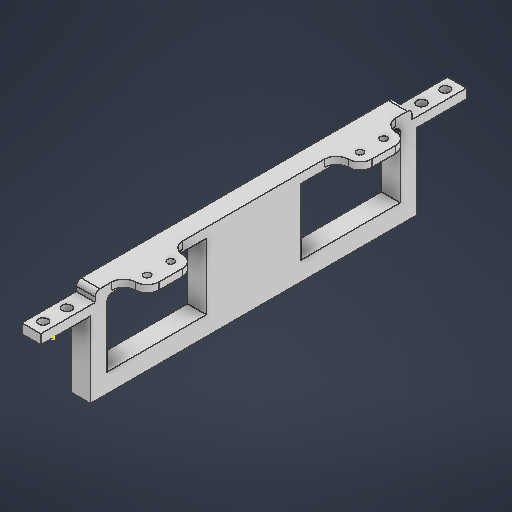
# Autodesk Inventor part: side_wall2
Saved by Autodesk Inventor 2026.1 (Build 301233000, 233)
## iProperties
Created: 2026-03-22
Part Number: side_wall2
Material: Generic
Document SubType Name: Modeling
Designer: emanuel
Density: 1 g/cm^3
Appearance: Default
Author: emanuel
Autodesk Inventor part; units mm, degrees
ref_plane "YZ Plane" through (0, 0, 0) normal (1, 0, 0) x (0, 1, 0)
ref_plane "XZ Plane" through (0, 0, 0) normal (0, 1, 0) x (-1, 0, 0)
ref_plane "XY Plane" through (0, 0, 0) normal (0, 0, 1) x (1, 0, 0)
sketch "Sketch1" plane through (0, 0, 0) normal (0, 1, 0) x (-1, 0, 0)
  circle A0 centre (0, 0) radius 2
  line L0 (0, 0) -> (0, -10)
  circle A1 centre (0, -10) radius 2
  line L1 (0, 0) -> (4, 0)
  line L2 (4, 0) -> (4, 5)
  line L3 (4, 5) -> (0, 5)
  line L4 (0, 5) -> (0, 0)
  line L5 (0, -10) -> (-4, -10)
  line L6 (-4, -10) -> (-4, -15)
  line L7 (-4, -15) -> (0, -15)
  line L8 (0, -15) -> (0, -10)
  line L9 (4, 5) -> (-4, 5)
  line L10 (-4, 5) -> (-4, -15)
  line L11 (-4, -15) -> (4, -15)
  line L12 (4, -15) -> (4, 5)
  line L13 (4, -15) -> (-4, -15)
  line L14 (-4, -15) -> (-4, -23)
  line L15 (-4, -23) -> (4, -23)
  line L16 (4, -23) -> (4, -15)
  line L17 (0, -10) -> (0, -85)
  line L18 (0, -85) -> (10, -85)
  circle A2 centre (0, -170) radius 2
  line L19 (0, -170) -> (0, -160)
  circle A3 centre (0, -160) radius 2
  line L20 (0, -170) -> (4, -170)
  line L21 (4, -170) -> (4, -175)
  line L22 (4, -175) -> (0, -175)
  line L23 (0, -175) -> (0, -170)
  line L24 (0, -160) -> (-4, -160)
  line L25 (-4, -160) -> (-4, -155)
  line L26 (-4, -155) -> (0, -155)
  line L27 (0, -155) -> (0, -160)
  line L28 (4, -175) -> (-4, -175)
  line L29 (-4, -175) -> (-4, -155)
  line L30 (-4, -155) -> (4, -155)
  line L31 (4, -155) -> (4, -175)
  line L32 (4, -155) -> (-4, -155)
  line L33 (-4, -155) -> (-4, -147)
  line L34 (-4, -147) -> (4, -147)
  line L35 (4, -147) -> (4, -155)
  dimension "d0" = 4
  dimension "d1" = 10
  dimension "d2" = 4
  dimension "d3" = 4
  dimension "d4" = 5
  dimension "d5" = 4
  dimension "d6" = 5
  dimension "d7" = 8
  dimension "d8" = 75
  dimension "d9" = 10
  constraints: 72 end point, 15 symmetric about line, 8 parallel, 5 perpendicular, 4 centre point, 4 coincident, 4 horizontal, 3 point on line, 1 vertical, 2 other
  measures "d0" diameter of A0
  measures "d1" distance of L0.start L0.end
  measures "d2" diameter of A1
  measures "d3" distance of L3.end L2.end
  measures "d4" distance of L2.end L1.end
  measures "d5" distance of L7.end L6.end
  measures "d6" distance of L6.end L5.end
  measures "d7" distance of L14.end L13.end
  measures "d8" distance of L5.start L17.end
  measures "d9" distance of L17.end L18.end
extrude "Extrusion1" add sketch "Sketch1" along normal blind 4 contours L1 L12 L11 L8 A1 L0 A0 | A0 L4 L3 L2 L1 | A0 L0 A1 L5 L10 L9 L4 | L16 L15 L17 L11 | A1 L8 L7 L6 L5 | L17 L15 L14 L7 | L20 L21 L22 L23 A2 | A2 L19 A3 L27 L30 L31 L20 | A2 L23 L28 L29 L24 A3 L19 | L30 L26 L33 L34 L35 | L24 L25 L26 L27 A3
sketch "Sketch2" plane through (0, 0, 0) normal (0, -1, 0) x (1, 0, 0)
  line L0 (4, -23) -> (-4, -23) projected
  line L1 (4, 5) -> (4, -23) projected
  line L2 (-4, -23) -> (4, -23)
  line L3 (4, -23) -> (4, -16)
  line L4 (4, -16) -> (-4, -16)
  line L5 (-4, -16) -> (-4, -23)
  line L6 (-4, -147) -> (4, -147) projected
  line L7 (-4, -147) -> (4, -147)
  line L8 (4, -147) -> (4, -154)
  line L9 (4, -154) -> (-4, -154)
  line L10 (-4, -154) -> (-4, -147)
  point P0 (0, 0)
  dimension "d12" = 7
  dimension "d13" = 7
  constraints: 16 end point, 4 parallel, 2 horizontal, 2 perpendicular, 2 point on line
  measures "d12" distance of L3.end L2.end
  measures "d13" distance of L7.end L8.end
extrude "Extrusion2" add sketch "Sketch2" along normal blind 32
sketch "Sketch3" plane through (0, -32, 0) normal (0, -1, 0) x (1, 0, 0)
  line L0 (4, -154) -> (4, -147) projected
  line L1 (-4, -16) -> (-4, -23) projected
  line L2 (4, -154) -> (-4, -154)
  line L3 (-4, -154) -> (-4, -16)
  line L4 (-4, -16) -> (4, -16)
  line L5 (4, -16) -> (4, -154)
  point P0 (0, 0)
  constraints: 8 end point, 2 parallel, 1 horizontal, 1 perpendicular
extrude "Extrusion3" add sketch "Sketch3" against normal blind 8
sketch "Sketch4" plane through (0, 4, 0) normal (0, 1, 0) x (1, 0, 0)
  line L0 (4, 23) -> (4, 147) projected
  line L1 (4, 147) -> (-4, 147)
  line L2 (-4, 147) -> (-4, 152)
  line L3 (-4, 152) -> (4, 152)
  line L4 (4, 152) -> (4, 147)
  line L5 (4, 23) -> (-4, 23) projected
  line L6 (4, 23) -> (-4, 23)
  line L7 (-4, 23) -> (-4, 18)
  line L8 (-4, 18) -> (4, 18)
  line L9 (4, 18) -> (4, 23)
  line L10 (-4, 18) -> (4, 18)
  line L11 (4, 18) -> (4, 152)
  line L12 (4, 152) -> (-4, 152)
  line L13 (-4, 152) -> (-4, 18)
  point P0 (0, 0)
  point P1 (-4, 23)
  dimension "d18" = 8
  dimension "d19" = 5
  dimension "d20" = 8
  dimension "d21" = 5
  constraints: 24 end point, 6 parallel, 3 horizontal, 3 perpendicular
  measures "d18" distance of L2.end L3.end
  measures "d19" distance of L1.end L2.end
  measures "d20" distance of L8.end L7.end
  measures "d21" distance of L7.end L6.end
extrude "Extrusion4" add sketch "Sketch4" along normal blind 4
sketch "Sketch5" plane through (0, -24, 0) normal (0, 1, 0) x (1, 0, 0)
  line L0 (4, 23) -> (-4, 23) projected
  line L1 (4, 23) -> (4, 147) projected
  line L2 (4, 23) -> (4, 147)
  line L3 (4, 85) -> (0, 85)
  line L4 (-4, 65) -> (4, 65)
  line L5 (4, 65) -> (4, 105)
  line L6 (4, 105) -> (-4, 105)
  line L7 (-4, 105) -> (-4, 65)
  line L8 (-4, 65) -> (4, 105) construction
  line L9 (4, 65) -> (-4, 105) construction
  point P0 (0, 0)
  point P1 (4, 65)
  point P2 (4, 105)
  dimension "d24" = 40
  constraints: 16 end point, 3 midpoint, 2 horizontal, 2 parallel, 1 perpendicular, 1 point on line, 1 vertical
  measures "d24" distance of L5.end L4.end
extrude "Extrusion5" add sketch "Sketch5" along normal up to surface (28 mm away)
fillet "Fillet1" radius 2 4 edges at (0, 4, -23) (0, 8, -18) (0, 8, -152) (0, 4, -147)
sketch "Sketch6" plane through (4, 0, 5) normal (1, 0, 0) x (0, 0, -1)
  point P0 (5, 0)
sketch "Sketch7" plane through (0, 8, 0) normal (0, 1, 0) x (1, 0, 0)
  line L0 (-4, 150) -> (4, 150) projected
  line L1 (4, 150) -> (4, 130)
  line L2 (4, 154) -> (4, 16) projected
  line L3 (4, 20) -> (-4, 20) projected
  line L4 (4, 20) -> (4, 40)
  line L5 (4, 130) -> (14, 130)
  line L6 (14, 130) -> (14, 120)
  line L7 (14, 120) -> (4, 120)
  line L8 (4, 120) -> (4, 130)
  line L9 (14, 130) -> (4, 130)
  line L10 (4, 130) -> (4, 140)
  line L11 (4, 140) -> (14, 140)
  line L12 (14, 140) -> (14, 130)
  line L13 (4, 40) -> (14, 40)
  line L14 (14, 40) -> (14, 50)
  line L15 (14, 50) -> (4, 50)
  line L16 (4, 50) -> (4, 40)
  line L17 (4, 40) -> (14, 40)
  line L18 (14, 40) -> (14, 30)
  line L19 (14, 30) -> (4, 30)
  line L20 (4, 30) -> (4, 40)
  line L21 (9, 40) -> (9, 45)
  line L22 (9, 40) -> (9, 35)
  circle A0 centre (9, 45) radius 1.5
  circle A1 centre (9, 35) radius 1.5
  line L23 (9, 130) -> (9, 135)
  line L24 (9, 130) -> (9, 125)
  circle A2 centre (9, 135) radius 1.5
  circle A3 centre (9, 125) radius 1.5
  point P0 (0, 0)
  dimension "d28" = 20
  dimension "d29" = 20
  dimension "d30" = 10
  dimension "d31" = 10
  dimension "d32" = 10
  dimension "d33" = 10
  dimension "d34" = 10
  dimension "d35" = 3
  dimension "d36" = 3
  dimension "d37" = 5
  dimension "d38" = 3
  dimension "d39" = 3
  constraints: 44 end point, 8 parallel, 4 centre point, 4 coincident, 4 horizontal, 4 perpendicular, 4 point on line, 4 vertical, 2 midpoint
  measures "d28" distance of L0.end L1.end
  measures "d29" distance of L3.start L4.end
  measures "d30" distance of L6.end L7.end
  measures "d31" distance of L5.end L6.end
  measures "d32" distance of L9.end L10.end
  measures "d33" distance of L15.end L14.end
  measures "d34" distance of L14.end L13.end
  measures "d35" diameter of A0
  measures "d36" diameter of A1
  measures "d37" distance of L23.start L23.end
  measures "d38" diameter of A2
  measures "d39" diameter of A3
extrude "Extrusion6" add sketch "Sketch7" against normal blind 3
fillet "Fillet2" radius 5 8 edges at (4, 6.5, -120) (14, 6.5, -120) (4, 6.5, -140) (14, 6.5, -140) (4, 6.5, -30) (14, 6.5, -30) (14, 6.5, -50) (4, 6.5, -50)
body "Solid1"
